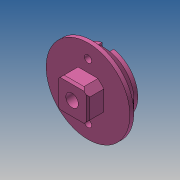
# Autodesk Inventor part: dado polea correa motor
Saved by Autodesk Inventor 2017 (Build 210142000, 142)
## iProperties
Part Number: dado polea correa motor
Material: Genérico
Document SubType Name: Modeling
Designer: Leo
Density: 1 g/cm^3
Appearance: Rosado
Description: Impresión 3d
Author: Leo
Autodesk Inventor part; units mm, degrees
ref_plane "YZ Plane" through (0, 0, 0) normal (1, 0, 0) x (0, 1, 0)
ref_plane "XZ Plane" through (0, 0, 0) normal (0, 1, 0) x (-1, 0, 0)
ref_plane "XY Plane" through (0, 0, 0) normal (0, 0, 1) x (1, 0, 0)
sketch "Boceto1" plane through (0, 0, 0) normal (0, 1, 0) x (-1, 0, 0)
  circle A0 centre (0, 0) radius 3.15
  circle A1 centre (0, 0) radius 15
  line L0 (-7.225, 3.7) -> (-10.925, 3.7)
  line L1 (-10.925, 3.7) -> (-10.925, -3.7)
  line L2 (-10.925, -3.7) -> (-7.225, -3.7)
  line L3 (-7.225, -3.7) -> (-7.225, 3.7)
  circle A2 centre (0, 0) radius 9.8003 construction
  point P0 (-7.225, 0)
  point P1 (-9.075, 3.7)
  dimension "d0" = 6.3
  dimension "tuerca" = 7.4
  dimension "d2" = 11.85
  dimension "d3" = 6.6503
  dimension "d4" = 3.7
  dimension "d26" = 30
  dimension "d27" = 4.075
  dimension "d28" = 4.075
  constraints: 8 end point, 2 centre point, 2 coincident, 2 midpoint, 2 parallel, 1 horizontal, 1 horizontal alignment, 1 perpendicular, 3 other
  measures "d0" diameter of A0
  measures "tuerca" distance of L0.end L1.end
  measures "d2" radial gap between concentric circles of A1 A0
  measures "d4" distance of L0.start L0.end
  measures "d26" diameter of A1
  measures "d27" distance edge to line of A0 L3
  measures "d28" distance edge to line of A1 L1
extrude "Extrusión1" add sketch "Boceto1" along normal blind 10
sketch "Boceto4" plane through (0, 0, 0) normal (1, 0, 0) x (0, 1, 0)
  line L0 (0, -15) -> (10, -15) projected
  line L1 (0, -15) -> (0, -21)
  line L2 (0, -21) -> (2, -21)
  line L3 (2, -21) -> (8, -15)
  line L4 (0, 0) -> (7.4976, 0)
  dimension "d47" = 45
  dimension "d48" = 21
  dimension "d49" = 2
  constraints: 8 end point, 2 horizontal, 1 point on line, 1 vertical
  measures "d47" angle of L0 L3
  measures "d48" distance from line of L4.start L2
  measures "d49" distance of L1.end L2.end
revolve "Revolución1" add sketch "Boceto4" angle 360 about axis through (0, 0, 0) along (0, 1, 0)
sketch "Boceto2" plane through (7.225, 0, -3.7) normal (1, 0, 0) x (0, 0, -1)
  line L0 (0, 0) -> (-7.4, 0) projected
  line L1 (0, 0) -> (0, 10) construction
  line L2 (-7.4, 10) -> (0, 10) construction
  line L3 (-7.4, 0) -> (-7.4, 10) construction
  line L4 (-7.4, 0) -> (0, 10) construction
  circle A0 centre (-3.7, 5) radius 2.1
  line L5 (0, 2.6329) -> (-4.5603, 0)
  line L6 (-2.8397, 0) -> (-7.4, 2.6329)
  line L7 (-7.4, 2.6329) -> (-7.4, 0)
  line L8 (0, 2.6329) -> (0, 0)
  point P0 (-3.7, 0)
  dimension "d7" = 4.2
  dimension "d8" = 120
  dimension "d9" = 3.9
  constraints: 10 end point, 4 point on line, 1 centre point, 1 collinear, 1 equal length, 1 horizontal alignment, 1 midpoint
  measures "d7" diameter of A0
  measures "d8" angle of L5 L6
  measures "d9" distance from line of A0.centre L5
extrude "Extrusión2" cut sketch "Boceto2" along normal mid plane 30 contours A0
extrude "Extrusión3" add sketch "Boceto2" along normal up to next contours L0 L6 L5 L8 | L0 L5 L6 | L0 L7 L6 L5
sketch "Boceto3" plane through (0, 0, 0) normal (0, -1, 0) x (1, 0, 0)
  circle A0 centre (0, 0) radius 3.15 projected
  circle A1 centre (0, 0) radius 27.5
  line L0 (-5, 8) -> (5, 8)
  line L1 (8, 5) -> (8, -5)
  line L2 (5, -8) -> (-5, -8)
  line L3 (-8, -5) -> (-8, 5)
  line L4 (-8, 5) -> (-5, 8)
  line L5 (5, 8) -> (8, 5)
  line L6 (8, -5) -> (5, -8)
  line L7 (-8, -5) -> (-5, -8)
  point P0 (-8, 8)
  point P1 (8, -8)
  point P2 (8, 8)
  point P3 (-8, -8)
  point P4 (-8, 0)
  point P5 (0, -8)
  dimension "d32" = 16
  dimension "d33" = 55
  dimension "d39" = 3
  dimension "d40" = 3
  dimension "d41" = 3
  dimension "d42" = 3
  dimension "d43" = 3
  dimension "d44" = 3
  dimension "d45" = 3
  dimension "d46" = 3
  constraints: 16 end point, 8 point on line, 2 midpoint, 2 parallel, 2 perpendicular, 1 centre point, 1 horizontal, 1 horizontal alignment, 1 vertical alignment
  measures "d32" distance of point (8, 8) point (8, -8)
  measures "d33" diameter of A1
  measures "d39" distance of L3.end point (-8, 8)
  measures "d40" distance of L0.start point (-8, 8)
  measures "d41" distance of L0.end point (8, 8)
  measures "d42" distance of L1.start point (8, 8)
  measures "d43" distance of L1.end point (8, -8)
  measures "d44" distance of L2.start point (8, -8)
  measures "d45" distance of L3.start point (-8, -8)
  measures "d46" distance of L2.end point (-8, -8)
extrude "Extrusión4" add sketch "Boceto3" along normal blind 8 contours L0 L5 L1 L6 L2 L7 L3 L4
chamfer "Chaflán1" distance 1 angle 45 4 edges at (9.075, 10, 3.7) (9.075, 10, -3.7) (10.925, 10, 0) (7.225, 10, 0)
chamfer "Chaflán3" distance 1 angle 45 4 edges at (0, -8, 8) (-8, -8, 0) (0, -8, -8) (8, -8, 0)
sketch "Boceto5" plane through (0, 10, 0) normal (0, 1, 0) x (1, 0, 0)
  line L0 (0, -14) -> (0, 14) construction
  point P0 (0, 0)
  point P1 (0, 0)
  dimension "d51" = 28
  constraints: 3 coincident, 2 end point, 1 midpoint, 1 vertical
  measures "d51" distance of L0.start L0.end
hole "Agujero1" at (0, 10, 14) at (0, 10, -14) direction (0, -1, 0) diameter 3.575 end through all counterbore diameter 6.5 counterbore depth 3
equation "\"d28\" = d27"
equation "\"d40\" = d39"
equation "\"d41\" = d39"
equation "\"d42\" = d41"
equation "\"d43\" = d39"
equation "\"d44\" = d43"
equation "\"d45\" = d39"
equation "\"d46\" = d45"
